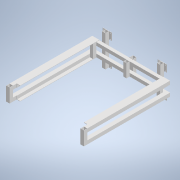
# Autodesk Inventor part: SoporteBobina
Saved by Autodesk Inventor 2020 (Build 240168000, 168)
## iProperties
Created: 2022-03-21
Part Number: SoporteBobina
Material: Genérico
Document SubType Name: Modeling
Designer: aarco
Density: 1 g/cm^3
Appearance: Valor por defecto
Mass: 5204.36 g
Surface Area: 21062.3 cm^2
Volume: 5204.36 cm^3
Author: aarco
Autodesk Inventor part; units mm, degrees
ref_plane "YZ Plane" through (0, 0, 0) normal (1, 0, 0) x (0, 1, 0)
ref_plane "XZ Plane" through (0, 0, 0) normal (0, 1, 0) x (-1, 0, 0)
ref_plane "XY Plane" through (0, 0, 0) normal (0, 0, 1) x (1, 0, 0)
sketch "Boceto1" plane through (0, 0, 0) normal (0, 0, 1) x (1, 0, 0)
  line L0 (0, 0) -> (-828.6689, 0) construction
  line L1 (0, 0) -> (821.843, 0) construction
  line L2 (-400, 150) -> (400, 150) construction
  line L3 (400, 150) -> (400, 0) construction
  line L4 (400, 0) -> (-400, 0) construction
  line L5 (-400, 0) -> (-400, 150) construction
  line L6 (0, 0) -> (0, 380.6015) construction
  line L7 (-404, 36) -> (-404, -4) construction
  line L8 (-404, -4) -> (-364, -4)
  line L9 (-364, -4) -> (-364, 0)
  line L10 (-364, 0) -> (-400, 0)
  line L11 (-400, 36) -> (-400, 0)
  line L12 (-404, 36) -> (-400, 36)
  line L13 (-404, -4) -> (-444, -4)
  line L14 (-444, -4) -> (-444, 36)
  line L15 (-444, 36) -> (-404, 36)
  line L16 (-404, 36) -> (-404, -4) construction
  line L17 (-442, 34) -> (-406, 34)
  line L18 (-406, 34) -> (-406, -2)
  line L19 (-406, -2) -> (-442, -2)
  line L20 (-442, -2) -> (-442, 34)
  line L21 (-424, 34) -> (-424, 36) construction
  line L22 (-442, 16) -> (-444, 16) construction
  line L23 (0, 0) -> (828.6689, 0) construction
  line L24 (0, 0) -> (-821.843, 0) construction
  line L25 (-400, 0) -> (400, 0) construction
  line L26 (404, 36) -> (404, -4) construction
  line L27 (404, -4) -> (364, -4)
  line L28 (364, -4) -> (364, 0)
  line L29 (364, 0) -> (400, 0)
  line L30 (400, 36) -> (400, 0)
  line L31 (404, 36) -> (400, 36)
  line L32 (404, -4) -> (444, -4)
  line L33 (444, -4) -> (444, 36)
  line L34 (444, 36) -> (404, 36)
  line L35 (404, 36) -> (404, -4) construction
  line L36 (442, 34) -> (406, 34)
  line L37 (406, 34) -> (406, -2)
  line L38 (406, -2) -> (442, -2)
  line L39 (442, -2) -> (442, 34)
  line L40 (424, 34) -> (424, 36) construction
  line L41 (442, 16) -> (444, 16) construction
  line L42 (400, 75) -> (-400, 75) construction
  line L43 (0, 150) -> (-828.6689, 150) construction
  line L44 (0, 150) -> (821.843, 150) construction
  line L45 (400, 150) -> (-400, 150) construction
  line L46 (0, 150) -> (0, -230.6015) construction
  line L47 (-404, 114) -> (-404, 154) construction
  line L48 (-404, 154) -> (-364, 154)
  line L49 (-364, 154) -> (-364, 150)
  line L50 (-364, 150) -> (-400, 150)
  line L51 (-400, 114) -> (-400, 150)
  line L52 (-404, 114) -> (-400, 114)
  line L53 (-404, 154) -> (-444, 154)
  line L54 (-444, 154) -> (-444, 114)
  line L55 (-444, 114) -> (-404, 114)
  line L56 (-404, 114) -> (-404, 154) construction
  line L57 (-442, 116) -> (-406, 116)
  line L58 (-406, 116) -> (-406, 152)
  line L59 (-406, 152) -> (-442, 152)
  line L60 (-442, 152) -> (-442, 116)
  line L61 (-424, 116) -> (-424, 114) construction
  line L62 (-442, 134) -> (-444, 134) construction
  line L63 (-400, 150) -> (400, 150) construction
  line L64 (364, 150) -> (400, 150)
  line L65 (364, 154) -> (364, 150)
  line L66 (404, 154) -> (364, 154)
  line L67 (0, 150) -> (828.6689, 150) construction
  line L68 (400, 114) -> (400, 150)
  line L69 (404, 114) -> (400, 114)
  line L70 (404, 114) -> (404, 154) construction
  line L71 (404, 114) -> (404, 154) construction
  line L72 (406, 116) -> (406, 152)
  line L73 (424, 116) -> (424, 114) construction
  line L74 (406, 152) -> (442, 152)
  line L75 (404, 154) -> (444, 154)
  line L76 (442, 152) -> (442, 116)
  line L77 (444, 154) -> (444, 114)
  line L78 (442, 134) -> (444, 134) construction
  line L79 (442, 116) -> (406, 116)
  line L80 (444, 114) -> (404, 114)
  line L81 (0, 150) -> (-821.843, 150) construction
  dimension "d0" = 800
  dimension "d1" = 150
  dimension "d3" = 4
  dimension "d5" = 40
  dimension "d7" = 40
  dimension "d8" = 2
  constraints: 164 end point, 60 symmetric about line, 12 perpendicular, 9 point on line, 6 midpoint, 6 parallel, 5 horizontal, 2 collinear, 2 vertical
  measures "d0" distance of L2.start L2.end
  measures "d1" distance of L4.end L2.start
  measures "d3" distance of L8.end L9.end
  measures "d5" distance between parallel lines of L8 L12
  measures "d7" distance of L13.end L14.end
  measures "d8" distance of L21.start L21.end
extrude "Extrusión1" add sketch "Boceto1" along normal blind 904
sketch "Boceto2" plane through (-400, 0, 0) normal (1, 0, 0) x (0, 0, -1)
  line L0 (0, 0) -> (0, 36) projected
  line L1 (0, 36) -> (-904, 36) projected
  line L2 (-904, 0) -> (-904, 36) projected
  line L3 (0, 0) -> (-904, 0) projected
  line L4 (0, 0) -> (0, 36) projected
  line L5 (0, 36) -> (-904, 36) projected
  line L6 (0, 0) -> (-36, 0)
  line L7 (-36, 0) -> (-36, 36)
  line L8 (-36, 36) -> (0, 36)
  line L9 (0, 36) -> (0, 0)
  line L10 (0, 114) -> (-904, 114) projected
  line L11 (0, 114) -> (-36, 114)
  line L12 (-36, 114) -> (-36, 150)
  line L13 (-36, 150) -> (0, 150)
  line L14 (0, 150) -> (0, 114)
  line L15 (0, 150) -> (-904, 150) projected
  constraints: 16 end point, 4 parallel, 4 perpendicular, 2 horizontal, 2 point on line
extrude "Extrusión2" add sketch "Boceto2" along normal up to next contours L3 L7 L1 L0 | L10 L12 L13 L14
sketch "Boceto10" plane through (0, 0, 904) normal (0, 0, 1) x (1, 0, 0)
  line L0 (-400, 114) -> (-400, 150) projected
  line L1 (-400, 150) -> (-364, 150) projected
  line L2 (-364, 150) -> (-364, 154) projected
  line L3 (-364, 154) -> (-444, 154) projected
  line L4 (-444, 154) -> (-444, 114) projected
  line L5 (-444, 114) -> (-400, 114) projected
  line L6 (-442, 152) -> (-406, 152) projected
  line L7 (-406, 152) -> (-406, 116) projected
  line L8 (-406, 116) -> (-442, 116) projected
  line L9 (-442, 116) -> (-442, 152) projected
  line L10 (-400, 36) -> (-444, 36) projected
  line L11 (-444, 36) -> (-444, -4) projected
  line L12 (-444, -4) -> (-364, -4) projected
  line L13 (-364, -4) -> (-364, 0) projected
  line L14 (-364, 0) -> (-400, 0) projected
  line L15 (-400, 0) -> (-400, 36) projected
  line L16 (-442, -2) -> (-442, 34) projected
  line L17 (-442, 34) -> (-406, 34) projected
  line L18 (-406, 34) -> (-406, -2) projected
  line L19 (-406, -2) -> (-442, -2) projected
  line L20 (400, 114) -> (444, 114) projected
  line L21 (444, 114) -> (444, 154) projected
  line L22 (444, 154) -> (364, 154) projected
  line L23 (364, 154) -> (364, 150) projected
  line L24 (364, 150) -> (400, 150) projected
  line L25 (400, 150) -> (400, 114) projected
  line L26 (442, 152) -> (442, 116) projected
  line L27 (442, 116) -> (406, 116) projected
  line L28 (406, 116) -> (406, 152) projected
  line L29 (406, 152) -> (442, 152) projected
  line L30 (400, 36) -> (400, 0) projected
  line L31 (400, 0) -> (364, 0) projected
  line L32 (364, 0) -> (364, -4) projected
  line L33 (364, -4) -> (444, -4) projected
  line L34 (444, -4) -> (444, 36) projected
  line L35 (444, 36) -> (400, 36) projected
  line L36 (442, 34) -> (442, -2) projected
  line L37 (442, -2) -> (406, -2) projected
  line L38 (406, -2) -> (406, 34) projected
  line L39 (406, 34) -> (442, 34) projected
  line L40 (-364, 154) -> (-444, 154) projected
  line L41 (-404, 154) -> (-404, -4)
  line L42 (-444, -4) -> (-364, -4) projected
  line L43 (404, -4) -> (404, 154)
  line L44 (444, 154) -> (364, 154) projected
  point P0 (0, 0)
  point P1 (404, 114)
  point P2 (404, 36)
  point P3 (-404, 114)
  point P4 (-404, -4)
  point P5 (-404, 36)
  dimension "d36" = 2
  dimension "d37" = 2
  constraints: 4 end point, 3 midpoint, 1 perpendicular, 1 vertical
  measures "d36" distance between parallel lines of L18 L41
  measures "d37" distance between parallel lines of L43 L28
extrude "Extrusión5" add sketch "Boceto10" along normal blind 40 contours L41 L12 L11 L10 | L5 L4 L3 L41 | L35 L34 L33 L43 | L43 L22 L21 L20
sketch "Boceto15" plane through (-444, -4, 0) normal (0, -1, 0) x (1, 0, 0)
  line L0 (0, 0) -> (0, 944) projected
  line L1 (0, 0) -> (40, 0)
  line L2 (40, 0) -> (40, -40)
  line L3 (40, -40) -> (0, -40)
  line L4 (0, -40) -> (0, 0)
  line L5 (888, 0) -> (848, 0)
  line L6 (848, 0) -> (848, -40)
  line L7 (848, -40) -> (888, -40)
  line L8 (888, -40) -> (888, 0)
  line L9 (2, -2) -> (38, -2)
  line L10 (38, -2) -> (38, -38)
  line L11 (38, -38) -> (2, -38)
  line L12 (2, -38) -> (2, -2)
  line L13 (2, -20) -> (0, -20) construction
  line L14 (20, -38) -> (20, -40) construction
  line L15 (850, -2) -> (886, -2)
  line L16 (886, -2) -> (886, -38)
  line L17 (886, -38) -> (850, -38)
  line L18 (850, -38) -> (850, -2)
  line L19 (848, -20) -> (850, -20) construction
  line L20 (868, -38) -> (868, -40) construction
  line L21 (424, 0) -> (464, 0)
  line L22 (464, 0) -> (464, -40)
  line L23 (464, -40) -> (424, -40)
  line L24 (424, -40) -> (424, 0)
  line L25 (426, -2) -> (462, -2)
  line L26 (462, -2) -> (462, -38)
  line L27 (462, -38) -> (426, -38)
  line L28 (426, -38) -> (426, -2)
  line L29 (424, -20) -> (426, -20) construction
  line L30 (444, -38) -> (444, -40) construction
  line L31 (808, 0) -> (888, 0) projected
  point P0 (444, 0)
  point P1 (444, 0)
  dimension "d46" = 40
  dimension "d47" = 2
  dimension "d48" = 2
  dimension "d51" = 2
  dimension "d52" = 40
  constraints: 60 end point, 13 midpoint, 12 parallel, 12 perpendicular, 7 equal length, 6 horizontal, 1 coincident
  measures "d46" distance of L3.end L0.start
  measures "d47" distance between parallel lines of L2 L10
  measures "d48" distance between parallel lines of L6 L18
  measures "d51" distance of L29.start L29.end
  measures "d52" distance of L23.end L21.start
extrude "Extrusión8" add sketch "Boceto15" against normal up to surface (158 mm away)
sketch "Boceto16" plane through (-364, -4, 0) normal (0, -1, 0) x (1, 0, 0)
  line L0 (-78, -38) -> (-78, -2) projected
  line L1 (-78, -2) -> (-42, -2) projected
  line L2 (-42, -2) -> (-42, -38) projected
  line L3 (-42, -38) -> (-78, -38) projected
  line L4 (-40, 0) -> (0, 0) projected
  line L5 (0, 0) -> (0, 904) projected
  line L6 (-40, 904) -> (0, 904) projected
  line L7 (-40, 904) -> (-40, 944) projected
  line L8 (-80, 944) -> (-40, 944) projected
  line L9 (-80, -40) -> (-80, 944) projected
  line L10 (-80, -40) -> (-40, -40) projected
  line L11 (-40, -40) -> (-40, 0) projected
  line L12 (770, -38) -> (770, -2) projected
  line L13 (770, -2) -> (806, -2) projected
  line L14 (806, -2) -> (806, -38) projected
  line L15 (806, -38) -> (770, -38) projected
  line L16 (728, 0) -> (768, 0) projected
  line L17 (768, 0) -> (768, -40) projected
  line L18 (768, -40) -> (808, -40) projected
  line L19 (808, -40) -> (808, 944) projected
  line L20 (768, 944) -> (808, 944) projected
  line L21 (768, 904) -> (768, 944) projected
  line L22 (728, 904) -> (768, 904) projected
  line L23 (728, 0) -> (728, 904) projected
  line L24 (-40, 0) -> (-80, 0) projected
  line L25 (-40, 0) -> (-80, 0)
  line L26 (-40, -40) -> (-40, 0) projected
  line L27 (-40, 0) -> (-80, 0)
  line L28 (768, 0) -> (728, 0) projected
  line L29 (768, 0) -> (808, 0) projected
  line L30 (768, 0) -> (808, 0)
  point P0 (364, 0)
  constraints: 6 end point, 3 collinear
extrude "Extrusión9" add sketch "Boceto16" along normal blind 100 contours L11 L10 L9 L24 | L29 L19 L18 L17
sketch "Boceto18" plane through (-400, 150, 904) normal (0, -1, 0) x (1, 0, 0)
  line L0 (0, -868) -> (0, 0) projected
  line L1 (36, -868) -> (36, 0) projected
  line L2 (0, -868) -> (36, -868)
  line L3 (36, -868) -> (36, -832)
  line L4 (36, -832) -> (0, -832)
  line L5 (0, -832) -> (0, -868)
  line L6 (764, -868) -> (800, -868) projected
  line L7 (764, -868) -> (764, 0) projected
  line L8 (800, -868) -> (764, -868)
  line L9 (764, -868) -> (764, -832)
  line L10 (764, -832) -> (800, -832)
  line L11 (800, -832) -> (800, -868)
  line L12 (36, -868) -> (764, -868) projected
  line L13 (382, -868) -> (418, -868)
  line L14 (418, -868) -> (418, -832)
  line L15 (418, -832) -> (382, -832)
  line L16 (382, -832) -> (382, -868)
  line L17 (384, -834) -> (416, -834)
  line L18 (416, -834) -> (416, -866)
  line L19 (416, -866) -> (384, -866)
  line L20 (384, -866) -> (384, -834)
  line L21 (400, -832) -> (400, -834) construction
  line L22 (384, -850) -> (382, -850) construction
  point P0 (400, -904)
  point P1 (400, -868)
  point P2 (0, -832)
  dimension "d55" = 2
  constraints: 36 end point, 9 perpendicular, 8 parallel, 6 midpoint, 5 point on line, 4 horizontal
  measures "d55" distance of L21.start L21.end
extrude "Extrusión10" add sketch "Boceto18" along normal up to surface (150 mm away)
sketch "Boceto19" plane through (364, 154, 904) normal (0, 1, 0) x (1, 0, 0)
  line L0 (42, 906) -> (78, 906) projected
  line L1 (42, 942) -> (42, 906) projected
  line L2 (78, 942) -> (42, 942) projected
  line L3 (78, 906) -> (78, 942) projected
  line L4 (40, 904) -> (0, 904) projected
  line L5 (0, 904) -> (0, 0) projected
  line L6 (40, 0) -> (0, 0) projected
  line L7 (40, 0) -> (40, -40) projected
  line L8 (80, -40) -> (40, -40) projected
  line L9 (80, 944) -> (80, -40) projected
  line L10 (40, 944) -> (80, 944) projected
  line L11 (40, 904) -> (40, 944) projected
  line L12 (-764, 868) -> (-728, 868) projected
  line L13 (-770, 904) -> (-770, -40) projected
  line L14 (-808, 944) -> (-808, -40) projected
  line L15 (-806, 906) -> (-770, 906) projected
  line L16 (-806, 942) -> (-806, 906) projected
  line L17 (-770, 942) -> (-806, 942) projected
  line L18 (-770, 906) -> (-770, 942) projected
  line L19 (-728, 904) -> (-768, 904) projected
  line L20 (-768, 944) -> (-768, 904) projected
  line L21 (-808, 944) -> (-768, 944) projected
  line L22 (-808, 944) -> (-808, -40) projected
  line L23 (-768, -40) -> (-808, -40) projected
  line L24 (-768, 0) -> (-768, -40) projected
  line L25 (-728, 0) -> (-768, 0) projected
  line L26 (-728, 904) -> (-728, 0) projected
  line L27 (-768, 944) -> (-768, 904) projected
  line L28 (-808, 904) -> (-768, 904) projected
  line L29 (-768, 904) -> (-808, 904)
  line L30 (40, 904) -> (80, 904) projected
  line L31 (40, 904) -> (80, 904)
  point P0 (-364, 904)
  constraints: 4 end point, 2 horizontal
extrude "Extrusión11" add sketch "Boceto19" along normal blind 100 contours L11 L10 L9 L30 | L28 L14 L21 L20
sketch "Boceto20" plane through (-404, -104, -40) normal (0, 0, -1) x (-1, 0, 0)
  line L0 (70, 0) -> (-30, 0)
  line L1 (-30, 0) -> (-30, 80)
  line L2 (-30, 80) -> (70, 80)
  line L3 (70, 80) -> (70, 0)
  line L4 (40, 0) -> (0, 0) projected
  line L5 (60, 10) -> (-20, 10) construction
  line L6 (-20, 10) -> (-20, 70) construction
  line L7 (-20, 70) -> (60, 70) construction
  line L8 (60, 70) -> (60, 10) construction
  line L9 (20, 0) -> (20, 10) construction
  line L10 (70, 40) -> (60, 40) construction
  circle A0 centre (60, 10) radius 5
  circle A1 centre (60, 70) radius 5
  circle A2 centre (-20, 70) radius 5
  circle A3 centre (-20, 10) radius 5
  line L11 (-384, 100) -> (-424, 100) construction
  line L12 (-404, 100) -> (-404, -48.3677) construction
  line L13 (38, 0) -> (38, 358) projected
  line L14 (38, 179) -> (218.9212, 179) construction
  line L15 (-878, 0) -> (-778, 0)
  line L16 (-778, 0) -> (-778, 80)
  line L17 (-778, 80) -> (-878, 80)
  line L18 (-878, 80) -> (-878, 0)
  line L19 (-848, 0) -> (-808, 0)
  line L20 (-868, 10) -> (-788, 10) construction
  line L21 (-788, 10) -> (-788, 70) construction
  line L22 (-788, 70) -> (-868, 70) construction
  line L23 (-868, 70) -> (-868, 10) construction
  line L24 (-828, 0) -> (-828, 10) construction
  line L25 (-878, 40) -> (-868, 40) construction
  circle A4 centre (-868, 10) radius 5
  circle A5 centre (-868, 70) radius 5
  circle A6 centre (-788, 70) radius 5
  circle A7 centre (-788, 10) radius 5
  line L26 (70, 358) -> (-30, 358)
  line L27 (-30, 358) -> (-30, 278)
  line L28 (-30, 278) -> (70, 278)
  line L29 (70, 278) -> (70, 358)
  line L30 (40, 358) -> (0, 358)
  line L31 (60, 348) -> (-20, 348) construction
  line L32 (-20, 348) -> (-20, 288) construction
  line L33 (-20, 288) -> (60, 288) construction
  line L34 (60, 288) -> (60, 348) construction
  line L35 (20, 358) -> (20, 348) construction
  line L36 (70, 318) -> (60, 318) construction
  circle A8 centre (60, 348) radius 5
  circle A9 centre (60, 288) radius 5
  circle A10 centre (-20, 288) radius 5
  circle A11 centre (-20, 348) radius 5
  line L37 (-384, 258) -> (-424, 258) construction
  line L38 (-404, 258) -> (-404, 406.3677) construction
  line L39 (-878, 318) -> (-868, 318) construction
  circle A12 centre (-868, 288) radius 5
  line L40 (-868, 288) -> (-868, 348) construction
  circle A13 centre (-868, 348) radius 5
  line L41 (-878, 278) -> (-878, 358)
  line L42 (-788, 288) -> (-868, 288) construction
  line L43 (-848, 358) -> (-808, 358)
  line L44 (-778, 278) -> (-878, 278)
  line L45 (-868, 348) -> (-788, 348) construction
  line L46 (-878, 358) -> (-778, 358)
  line L47 (-828, 358) -> (-828, 348) construction
  line L48 (-788, 348) -> (-788, 288) construction
  line L49 (-778, 358) -> (-778, 278)
  circle A14 centre (-788, 288) radius 5
  circle A15 centre (-788, 348) radius 5
  point P0 (-404, 104)
  point P1 (-846, 0)
  point P2 (-404, 254)
  point P3 (-846, 358)
  dimension "d60" = 100
  dimension "d61" = 80
  dimension "d62" = 80
  dimension "d63" = 60
  dimension "d64" = 10
  dimension "d65" = 10
  dimension "d66" = 10
  dimension "d67" = 10
  constraints: 94 end point, 61 symmetric about line, 16 centre point, 16 coincident, 7 midpoint, 4 parallel, 4 perpendicular, 3 horizontal, 1 vertical, 12 other
  measures "d60" distance of L0.start L0.end
  measures "d61" distance of L2.end L0.start
  measures "d62" distance of L5.start L5.end
  measures "d63" distance of L5.end L6.end
  measures "d64" diameter of A0
  measures "d65" diameter of A1
  measures "d66" diameter of A2
  measures "d67" diameter of A3
extrude "Extrusión12" add sketch "Boceto20" along normal blind 3
sketch "Boceto22" plane through (364, 154, 904) normal (0, 1, 0) x (1, 0, 0)
  line L0 (40, -40) -> (80, -40) projected
  line L1 (80, -40) -> (40, -40)
  line L2 (40, -40) -> (40, -80)
  line L3 (40, -80) -> (80, -80)
  line L4 (80, -80) -> (80, -40)
  line L5 (-808, 904) -> (-808, -40) projected
  line L6 (-808, -40) -> (-768, -40)
  line L7 (-768, -40) -> (-768, -80)
  line L8 (-768, -80) -> (-808, -80)
  line L9 (-808, -80) -> (-808, -40)
  line L10 (78, -78) -> (42, -78)
  line L11 (42, -78) -> (42, -42)
  line L12 (42, -42) -> (78, -42)
  line L13 (78, -42) -> (78, -78)
  line L14 (60, -78) -> (60, -80) construction
  line L15 (78, -60) -> (80, -60) construction
  line L16 (-770, -78) -> (-806, -78)
  line L17 (-806, -78) -> (-806, -42)
  line L18 (-806, -42) -> (-770, -42)
  line L19 (-770, -42) -> (-770, -78)
  line L20 (-788, -78) -> (-788, -80) construction
  line L21 (-770, -60) -> (-768, -60) construction
  point P0 (-364, 904)
  dimension "d70" = 40
  dimension "d71" = 2
  dimension "d72" = 2
  constraints: 40 end point, 12 perpendicular, 8 midpoint, 8 parallel, 4 horizontal, 1 coincident
  measures "d70" distance of L2.end L3.end
  measures "d71" distance between parallel lines of L9 L17
  measures "d72" distance between parallel lines of L4 L13
extrude "Extrusión13" add sketch "Boceto22" against normal up to surface (158 mm away)
sketch "Boceto23" plane through (-364, 150, 36) normal (0, 1, 0) x (1, 0, 0)
  line L0 (384, 36) -> (728, 36) projected
  line L1 (698, 36) -> (658, 36)
  line L2 (658, 36) -> (658, 76)
  line L3 (658, 76) -> (698, 76)
  line L4 (698, 76) -> (698, 36)
  line L5 (808, 36) -> (808, 76) projected
  line L6 (728, 76) -> (628, 76) construction
  line L7 (628, 76) -> (628, 79) construction
  line L8 (628, 79) -> (728, 79) construction
  line L9 (728, 79) -> (728, 76) construction
  line L10 (738, 79) -> (838, 79) projected
  line L11 (738, 76) -> (738, 79) projected
  line L12 (364, 36) -> (364, 158.6552) construction
  line L13 (696, 38) -> (660, 38)
  line L14 (660, 38) -> (660, 74)
  line L15 (660, 74) -> (696, 74)
  line L16 (696, 74) -> (696, 38)
  line L17 (678, 38) -> (678, 36) construction
  line L18 (696, 56) -> (698, 56) construction
  line L19 (30, 36) -> (70, 36)
  line L20 (70, 36) -> (70, 76)
  line L21 (70, 76) -> (30, 76)
  line L22 (30, 76) -> (30, 36)
  line L23 (0, 76) -> (100, 76) construction
  line L24 (100, 76) -> (100, 79) construction
  line L25 (100, 79) -> (0, 79) construction
  line L26 (0, 79) -> (0, 76) construction
  line L27 (32, 38) -> (68, 38)
  line L28 (68, 38) -> (68, 74)
  line L29 (68, 74) -> (32, 74)
  line L30 (32, 74) -> (32, 38)
  line L31 (50, 38) -> (50, 36) construction
  line L32 (32, 56) -> (30, 56) construction
  point P0 (678, 76)
  point P1 (0, 36)
  point P2 (-10, 79)
  point P3 (50, 76)
  point P4 (-10, 76)
  dimension "d75" = 10
  dimension "d76" = 2
  constraints: 58 end point, 20 symmetric about line, 6 midpoint, 6 parallel, 5 equal length, 5 perpendicular, 3 horizontal, 1 point on line, 1 vertical
  measures "d75" distance between parallel lines of L11 L9
  measures "d76" distance between parallel lines of L4 L16
extrude "Extrusión14" add sketch "Boceto23" against normal up to surface (150 mm away)
sketch "Boceto24" plane through (-364, 150, 36) normal (0, 1, 0) x (1, 0, 0)
  line L0 (698, 36) -> (658, 36)
  line L1 (70, 36) -> (30, 36)
  line L2 (698, 36) -> (698, 76) projected
  line L3 (696, 74) -> (696, 38) projected
  line L4 (698, 76) -> (658, 76) projected
  line L5 (660, 74) -> (696, 74) projected
  line L6 (660, 38) -> (660, 74) projected
  line L7 (658, 76) -> (658, 36) projected
  line L8 (30, 76) -> (30, 36) projected
  line L9 (32, 38) -> (32, 74) projected
  line L10 (70, 76) -> (30, 76) projected
  line L11 (70, 36) -> (70, 76) projected
  line L12 (68, 74) -> (68, 38) projected
  line L13 (32, 74) -> (68, 74) projected
  line L14 (696, 38) -> (660, 38) projected
  line L15 (68, 38) -> (32, 38) projected
  point P0 (364, 36)
  constraints: 4 end point, 2 horizontal
extrude "Extrusión15" add sketch "Boceto24" along normal up to surface (104 mm away)
sketch "Boceto25" plane through (364, 0, 0) normal (0, -1, 0) x (1, 0, 0)
  line L0 (-30, -40) -> (-30, 0) projected
  line L1 (-70, -40) -> (-30, -40) projected
  line L2 (-70, 0) -> (-70, -40) projected
  line L3 (-30, 0) -> (-70, 0) projected
  line L4 (-32, -38) -> (-68, -38) projected
  line L5 (-32, -2) -> (-32, -38) projected
  line L6 (-68, -2) -> (-32, -2) projected
  line L7 (-68, -38) -> (-68, -2) projected
  line L8 (-660, -2) -> (-660, -38) projected
  line L9 (-696, -2) -> (-660, -2) projected
  line L10 (-696, -38) -> (-696, -2) projected
  line L11 (-660, -38) -> (-696, -38) projected
  line L12 (-698, -40) -> (-658, -40) projected
  line L13 (-698, 0) -> (-698, -40) projected
  line L14 (-658, 0) -> (-698, 0) projected
  line L15 (-658, -40) -> (-658, 0) projected
  point P0 (-364, 0)
extrude "Extrusión16" add sketch "Boceto25" along normal up to surface (104 mm away)
sketch "Boceto26" plane through (-294, 254, -40) normal (0, 0, -1) x (-1, 0, 0)
  line L0 (-658, -278) -> (-558, -278)
  line L1 (-558, -278) -> (-558, -358)
  line L2 (-558, -358) -> (-658, -358)
  line L3 (-658, -358) -> (-658, -278)
  line L4 (-668, -278) -> (-698, -278) projected
  line L5 (-668, -278) -> (-658, -278) construction
  line L6 (-668, -358) -> (-668, -278) projected
  line L7 (-768, -358) -> (-668, -358) projected
  line L8 (-628, -358) -> (-588, -358) projected
  line L9 (-663, -278) -> (-663, -386.9665) construction
  circle A0 centre (-678, -288) radius 5 projected
  circle A1 centre (-678, -348) radius 5 projected
  circle A2 centre (-758, -348) radius 5 projected
  circle A3 centre (-758, -288) radius 5 projected
  circle A4 centre (-648, -288) radius 5
  circle A5 centre (-648, -348) radius 5
  circle A6 centre (-568, -348) radius 5
  circle A7 centre (-568, -288) radius 5
  line L10 (-314, -258) -> (-274, -258) projected
  line L11 (-294, -258) -> (-294, -515.9052)
  line L12 (-314, -218) -> (-314, -140) projected
  line L13 (-314, -179) -> (-941.3867, -179)
  line L14 (70, -278) -> (-30, -278)
  line L15 (-30, -278) -> (-30, -358)
  line L16 (-30, -358) -> (70, -358)
  line L17 (70, -358) -> (70, -278)
  line L18 (80, -278) -> (70, -278) construction
  line L19 (40, -358) -> (0, -358)
  circle A8 centre (60, -288) radius 5
  circle A9 centre (-20, -288) radius 5
  circle A10 centre (-20, -348) radius 5
  circle A11 centre (60, -348) radius 5
  line L20 (-658, -80) -> (-558, -80)
  line L21 (-558, -80) -> (-558, 0)
  line L22 (-558, 0) -> (-658, 0)
  line L23 (-658, 0) -> (-658, -80)
  line L24 (-668, -80) -> (-658, -80) construction
  line L25 (-628, 0) -> (-588, 0)
  line L26 (-663, -80) -> (-663, 28.9665) construction
  circle A12 centre (-648, -70) radius 5
  circle A13 centre (-568, -70) radius 5
  circle A14 centre (-568, -10) radius 5
  circle A15 centre (-648, -10) radius 5
  line L27 (-314, -100) -> (-274, -100)
  line L28 (-294, -100) -> (-294, 157.9052)
  line L29 (70, 0) -> (70, -80)
  line L30 (80, -80) -> (70, -80) construction
  circle A16 centre (60, -70) radius 5
  circle A17 centre (60, -10) radius 5
  circle A18 centre (-20, -70) radius 5
  line L31 (40, 0) -> (0, 0)
  circle A19 centre (-20, -10) radius 5
  line L32 (70, -80) -> (-30, -80)
  line L33 (-30, -80) -> (-30, 0)
  line L34 (-30, 0) -> (70, 0)
  point P0 (-294, -254)
  point P1 (-608, -358)
  point P2 (20, -358)
  point P3 (-294, -104)
  point P4 (-608, 0)
  point P5 (20, 0)
  point P6 (0, -358)
  point P7 (40, -358)
  point P8 (40, 0)
  point P9 (0, 0)
  constraints: 58 end point, 47 symmetric about line, 16 centre point, 5 midpoint, 2 equal length, 2 horizontal, 2 parallel, 2 perpendicular, 2 vertical, 16 other
extrude "Extrusión17" add sketch "Boceto26" along normal up to surface (3 mm away) contours L0 L1 L2 L3 | L17 L16 L15 L14 | L23 L22 L21 L20 | L29 L32 L33 L34 L31
sketch "Boceto28" plane through (-404, -104, -43) normal (0, 0, -1) x (-1, 0, 0)
  line L0 (0, 100) -> (-40, 100) projected
  line L1 (113.3047, -17.5248) -> (-31.6838, -17.5248)
  line L2 (-31.6838, -17.5248) -> (-31.6838, 100)
  line L3 (-31.6838, 100) -> (113.3047, 100)
  line L4 (113.3047, 100) -> (113.3047, -17.5248)
  line L5 (-40, 258) -> (0, 258) projected
  line L6 (-35.6215, 258) -> (89.8114, 258)
  line L7 (89.8114, 258) -> (89.8114, 377.7923)
  line L8 (89.8114, 377.7923) -> (-35.6215, 377.7923)
  line L9 (-35.6215, 377.7923) -> (-35.6215, 258)
  line L10 (-808, 258) -> (-768, 258) projected
  line L11 (-775.4059, 258) -> (-948.375, 258)
  line L12 (-948.375, 258) -> (-948.375, 373.3298)
  line L13 (-948.375, 373.3298) -> (-775.4059, 373.3298)
  line L14 (-775.4059, 373.3298) -> (-775.4059, 258)
  line L15 (-768, 100) -> (-808, 100) projected
  line L16 (-772.0661, 100) -> (-901.994, 100)
  line L17 (-901.994, 100) -> (-901.994, -48.91)
  line L18 (-901.994, -48.91) -> (-772.0661, -48.91)
  line L19 (-772.0661, -48.91) -> (-772.0661, 100)
  line L20 (-891.3544, -17.5248) -> (-795.4538, -17.5248)
  line L21 (-795.4538, -17.5248) -> (-795.4538, 327.1008)
  line L22 (-795.4538, 327.1008) -> (-891.3544, 327.1008)
  line L23 (-891.3544, 327.1008) -> (-891.3544, -17.5248)
  line L24 (-11.8018, 59.1377) -> (78.1063, 59.1377)
  line L25 (78.1063, 59.1377) -> (78.1063, 341.1922)
  line L26 (78.1063, 341.1922) -> (-11.8018, 341.1922)
  line L27 (-11.8018, 341.1922) -> (-11.8018, 59.1377)
  point P0 (-404, 104)
  point P1 (-11.8018, 258)
  point P2 (-11.8018, 100)
  point P3 (78.1063, 100)
  point P4 (78.1063, 258)
  point P5 (-891.3544, 258)
  point P6 (-891.3544, 100)
  point P7 (-795.4538, 100)
  point P8 (-795.4538, 258)
  constraints: 48 end point, 12 parallel, 6 horizontal, 6 perpendicular, 4 point on line
extrude "Extrusión18" cut sketch "Boceto28" against normal up to surface (43 mm away)
